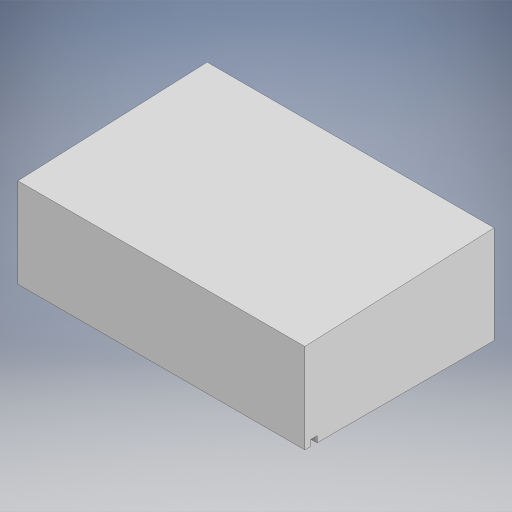
# Autodesk Inventor part: Part1
Saved by Autodesk Inventor 2023.1 (Build 271208000, 208)
## iProperties
Created: 2022-10-28
Part Number: Part1
Material: Generic
Document SubType Name: Modeling
Designer: awelt
Mass: 19265.3 g
Surface Area: 4898.59 cm^2
Volume: 19265.3 cm^3
Density: 1 g/cm^3
Appearance: Default
Author: awelt
Autodesk Inventor part; units mm, degrees
ref_plane "YZ Plane" through (0, 0, 0) normal (1, 0, 0) x (0, 1, 0)
ref_plane "XZ Plane" through (0, 0, 0) normal (0, 1, 0) x (-1, 0, 0)
ref_plane "XY Plane" through (0, 0, 0) normal (0, 0, 1) x (1, 0, 0)
sketch "Sketch1" plane through (0, 0, 0) normal (1, 0, 0) x (0, 1, 0)
  line L0 (0, 0) -> (152.4, 0)
  line L1 (152.4, 0) -> (152.4, -295.275)
  line L2 (152.4, -295.275) -> (0, -295.275)
  line L3 (0, -295.275) -> (0, 0)
  line L4 (152.4, -295.275) -> (139.7, 0)
  line L5 (0, -9.525) -> (9.525, -9.525)
  line L6 (9.525, -9.525) -> (9.525, -19.05)
  line L7 (9.525, -19.05) -> (0, -19.05)
  line L8 (0, -19.05) -> (0, -9.525)
  point P0 (0, -19.05)
  dimension "d0" = 152.4
  dimension "d1" = 295.275
  dimension "d2" = 12.7
  dimension "d3" = 9.525
  dimension "d4" = 9.525
  dimension "d5" = 9.525
  constraints: 18 end point, 4 parallel, 2 horizontal, 2 perpendicular, 2 point on line
  measures "d0" distance of L1.end L2.end
  measures "d1" distance of L0.end L1.end
  measures "d2" distance of L4.end L0.end
  measures "d3" distance of L6.end L7.end
  measures "d4" distance of L5.end L6.end
  measures "d5" distance of L5.start L0.start
extrude "Extrusion1" add sketch "Sketch1" along normal blind 447.675 contours L0 L4 L2 L3 L7 L6 L5
equation "\"d5\" = d3"
body "Solid1"
